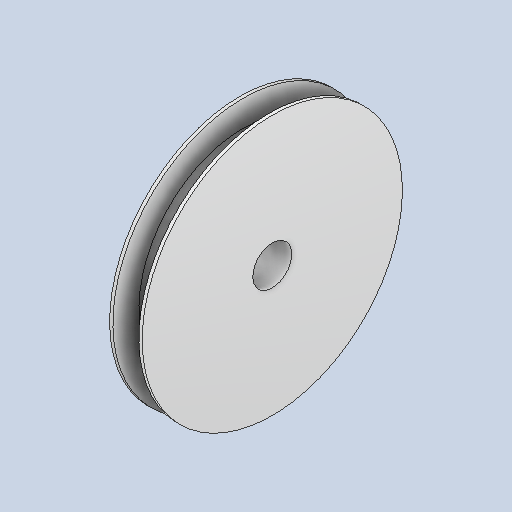
# Autodesk Inventor part: Zugscheibe_für_Kette
Saved by Autodesk Inventor 2025.2 (Build 292293000, 293)
## iProperties
Created: 2025-02-03
Part Number: Zugscheibe_für_Kette
Material: Generisch
Document SubType Name: Modeling
Designer: unter
Density: 1 g/cm^3
Appearance: Blau-Gelb
Author: unter
Autodesk Inventor part; units mm, degrees
ref_plane "YZ Plane" through (0, 0, 0) normal (1, 0, 0) x (0, 1, 0)
ref_plane "XZ Plane" through (0, 0, 0) normal (0, 1, 0) x (-1, 0, 0)
ref_plane "XY Plane" through (0, 0, 0) normal (0, 0, 1) x (1, 0, 0)
derived "Skelett_Laufkatze.ipt"
sketch "Kettenzug_scheibe_front" plane through (-208, 0, 62.4) normal (-1, 0, 0) x (0, -1, 0)
  line L0 (-15, 0) -> (0, 0)
  circle A0 centre (0, 0) radius 15
  circle A1 centre (0, 0) radius 100
  point P0 (0, -62.4)
sketch "Kettenzug_scheibe_seite" plane through (-131, 0, 62.4) normal (0, 0, -1) x (-1, 0, 0)
  line L0 (77, 0) -> (52, 0)
  line L1 (77, 15) -> (52, 15)
  line L2 (52, 15) -> (52, 100)
  line L3 (77, 100) -> (77, 15)
  line L4 (74.5, 100) -> (74.5, 80)
  line L5 (74.5, 80) -> (54.5, 80)
  line L6 (54.5, 80) -> (54.5, 100)
  line L7 (64.5, 100) -> (64.5, 80) construction
  line L8 (77, 100) -> (74.5, 100)
  line L9 (54.5, 100) -> (52, 100)
  line L10 (74.5, 100) -> (54.5, 100) construction
  point P0 (-131, 0)
revolve "Rohling_Scheibe" add sketch "Kettenzug_scheibe_seite" angle 360 about axis through (-208, 0, 62.4) along (1, 0, 0)
